Autodesk Inventor part; units mm, degrees
(part 4 of 4)
  spline S763 degree 2 poles (254.6918, 603.0222) (254.6054, 602.9877) (254.4448, 602.8889) (254.3954, 602.8543) knots 0 0 0 1 2 2 2
  line L811 (254.3954, 602.8543) -> (254.3732, 602.8543)
  line L812 (254.3732, 602.8543) -> (254.3732, 603.289)
  spline S764 degree 2 poles (254.3732, 603.289) (254.4991, 603.3508) (254.9512, 603.4718) (255.1537, 603.4718) knots 0 0 0 1 2 2 2
  spline S765 degree 2 poles (255.1537, 603.4718) (255.581, 603.4718) (256.0627, 603.0198) (256.0627, 602.6344) knots 0 0 0 1 2 2 2
  spline S766 degree 2 poles (256.0627, 602.6344) (256.0627, 602.4541) (255.9787, 602.1528) (255.9046, 602.0244) knots 0 0 0 1 2 2 2
  spline S767 degree 2 poles (255.9046, 602.0244) (255.8305, 601.891) (255.6156, 601.6292) (255.497, 601.5032) knots 0 0 0 1 2 2 2
  spline S768 degree 2 poles (255.497, 601.5032) (255.3044, 601.2932) (254.8326, 600.8437) (254.6918, 600.7128) knots 0 0 0 1 2 2 2
  line L813 (254.6918, 600.7128) -> (256.1886, 600.7128)
  line L814 (256.1886, 600.7128) -> (256.1886, 600.3596)
  line L815 (259.3305, 600.3596) -> (258.8068, 600.3596)
  line L816 (258.8068, 600.3596) -> (258.3894, 600.7968)
  spline S769 degree 2 poles (258.3894, 600.7968) (258.1819, 600.53) (257.7423, 600.2953) (257.4632, 600.2953) knots 0 0 0 1 2 2 2
  spline S770 degree 2 poles (257.4632, 600.2953) (257.0507, 600.2953) (256.5122, 600.7943) (256.5122, 601.1969) knots 0 0 0 1 2 2 2
  spline S771 degree 2 poles (256.5122, 601.1969) (256.5122, 601.3723) (256.611, 601.6464) (256.6925, 601.7576) knots 0 0 0 1 2 2 2
  spline S772 degree 2 poles (256.6925, 601.7576) (256.7716, 601.8638) (256.9815, 602.0268) (257.0754, 602.0861) knots 0 0 0 1 2 2 2
  spline S773 degree 2 poles (257.0754, 602.0861) (256.8704, 602.2244) (256.6653, 602.5332) (256.6653, 602.7654) knots 0 0 0 1 2 2 2
  spline S774 degree 2 poles (256.6653, 602.7654) (256.6653, 602.9111) (256.7814, 603.1581) (256.8753, 603.252) knots 0 0 0 1 2 2 2
  spline S775 degree 2 poles (256.8753, 603.252) (256.9741, 603.3483) (257.2878, 603.4718) (257.473, 603.4718) knots 0 0 0 1 2 2 2
  spline S776 degree 2 poles (257.473, 603.4718) (257.8139, 603.4718) (258.2437, 603.1136) (258.2437, 602.8395) knots 0 0 0 1 2 2 2
  spline S777 degree 2 poles (258.2437, 602.8395) (258.2437, 602.7382) (258.1918, 602.5233) (258.1251, 602.4245) knots 0 0 0 1 2 2 2
  spline S778 degree 2 poles (258.1251, 602.4245) (258.056, 602.3232) (257.8386, 602.1479) (257.6558, 602.0812) knots 0 0 0 1 2 2 2
  line L817 (257.6558, 602.0812) -> (258.3746, 601.3402)
  spline S779 degree 2 poles (258.3746, 601.3402) (258.4018, 601.5081) (258.4141, 601.9033) (258.4141, 602.222) knots 0 0 0 1 2 2 2
  line L818 (258.4141, 602.222) -> (258.8143, 602.222)
  line L819 (258.8143, 602.222) -> (258.8143, 602.0244)
  spline S780 degree 2 poles (258.8143, 602.0244) (258.8143, 601.8292) (258.7155, 601.3352) (258.5994, 601.1129) knots 0 0 0 1 2 2 2
  line L820 (258.5994, 601.1129) -> (259.3305, 600.3596)
  line L821 (258.2116, 600.9771) -> (257.2705, 601.9404)
  spline S781 degree 2 poles (257.2705, 601.9404) (257.2211, 601.9083) (257.1198, 601.8169) (257.0581, 601.728) knots 0 0 0 1 2 2 2
  spline S782 degree 2 poles (257.0581, 601.728) (257.0087, 601.6563) (256.9346, 601.4241) (256.9346, 601.2957) knots 0 0 0 1 2 2 2
  spline S783 degree 2 poles (256.9346, 601.2957) (256.9346, 601.0042) (257.2804, 600.6288) (257.5743, 600.6288) knots 0 0 0 1 2 2 2
  spline S784 degree 2 poles (257.5743, 600.6288) (257.7694, 600.6288) (258.0831, 600.7943) (258.2116, 600.9771) knots 0 0 0 1 2 2 2
  spline S785 degree 2 poles (257.4632, 602.2269) (257.5768, 602.2664) (257.7275, 602.3973) (257.7694, 602.4739) knots 0 0 0 1 2 2 2
  spline S786 degree 2 poles (257.7694, 602.4739) (257.8065, 602.5455) (257.8435, 602.7061) (257.8435, 602.7999) knots 0 0 0 1 2 2 2
  spline S787 degree 2 poles (257.8435, 602.7999) (257.8435, 602.9975) (257.6114, 603.2149) (257.4582, 603.2149) knots 0 0 0 1 2 2 2
  spline S788 degree 2 poles (257.4582, 603.2149) (257.2754, 603.2149) (257.0655, 602.9679) (257.0655, 602.7851) knots 0 0 0 1 2 2 2
  spline S789 degree 2 poles (257.0655, 602.7851) (257.0655, 602.7036) (257.0951, 602.585) (257.1445, 602.5085) knots 0 0 0 1 2 2 2
  spline S790 degree 2 poles (257.1445, 602.5085) (257.189, 602.4443) (257.3421, 602.301) (257.4632, 602.2269) knots 0 0 0 1 2 2 2
  spline S791 degree 2 poles (260.0937, 600.3052) (259.864, 600.3052) (259.4663, 600.4287) (259.3354, 600.4979) knots 0 0 0 1 2 2 2
  line L822 (259.3354, 600.4979) -> (259.3354, 600.9301)
  line L823 (259.3354, 600.9301) -> (259.3552, 600.9301)
  spline S792 degree 2 poles (259.3552, 600.9301) (259.4046, 600.8906) (259.538, 600.7968) (259.6491, 600.7449) knots 0 0 0 1 2 2 2
  spline S793 degree 2 poles (259.6491, 600.7449) (259.7455, 600.698) (259.9826, 600.6288) (260.1085, 600.6288) knots 0 0 0 1 2 2 2
  spline S794 degree 2 poles (260.1085, 600.6288) (260.1999, 600.6288) (260.4099, 600.6708) (260.4593, 600.7054) knots 0 0 0 1 2 2 2
  spline S795 degree 2 poles (260.4593, 600.7054) (260.5309, 600.7523) (260.5951, 600.8585) (260.5951, 600.9672) knots 0 0 0 1 2 2 2
  spline S796 degree 2 poles (260.5951, 600.9672) (260.5951, 601.103) (260.4469, 601.2438) (260.2567, 601.2908) knots 0 0 0 1 2 2 2
  spline S797 degree 2 poles (260.2567, 601.2908) (260.1826, 601.3081) (259.9455, 601.3575) (259.8443, 601.3846) knots 0 0 0 1 2 2 2
  spline S798 degree 2 poles (259.8443, 601.3846) (259.5824, 601.4612) (259.3453, 601.7774) (259.3453, 602.0021) knots 0 0 0 1 2 2 2
  spline S799 degree 2 poles (259.3453, 602.0021) (259.3453, 602.3133) (259.8121, 602.7011) (260.1975, 602.7011) knots 0 0 0 1 2 2 2
  spline S800 degree 2 poles (260.1975, 602.7011) (260.3877, 602.7011) (260.773, 602.6073) (260.9039, 602.5356) knots 0 0 0 1 2 2 2
  line L824 (260.9039, 602.5356) -> (260.9039, 602.1232)
  line L825 (260.9039, 602.1232) -> (260.8841, 602.1232)
  spline S801 degree 2 poles (260.8841, 602.1232) (260.7359, 602.2417) (260.3753, 602.3776) (260.1901, 602.3776) knots 0 0 0 1 2 2 2
  spline S802 degree 2 poles (260.1901, 602.3776) (259.9999, 602.3776) (259.738, 602.217) (259.738, 602.0565) knots 0 0 0 1 2 2 2
  spline S803 degree 2 poles (259.738, 602.0565) (259.738, 601.9107) (259.8937, 601.7699) (260.0666, 601.7255) knots 0 0 0 1 2 2 2
  spline S804 degree 2 poles (260.0666, 601.7255) (260.1505, 601.7033) (260.363, 601.6588) (260.479, 601.6316) knots 0 0 0 1 2 2 2
  spline S805 degree 2 poles (260.479, 601.6316) (260.731, 601.5674) (260.9879, 601.2735) (260.9879, 601.0191) knots 0 0 0 1 2 2 2
  spline S806 degree 2 poles (260.9879, 601.0191) (260.9879, 600.8709) (260.8718, 600.609) (260.7582, 600.5127) knots 0 0 0 1 2 2 2
  spline S807 degree 2 poles (260.7582, 600.5127) (260.6371, 600.4114) (260.3284, 600.3052) (260.0937, 600.3052) knots 0 0 0 1 2 2 2
  line L826 (262.5588, 602.2343) -> (262.539, 602.2343)
  spline S808 degree 2 poles (262.539, 602.2343) (262.4946, 602.2467) (262.3983, 602.2516) (262.3316, 602.2516) knots 0 0 0 1 2 2 2
  spline S809 degree 2 poles (262.3316, 602.2516) (262.176, 602.2516) (261.8697, 602.1157) (261.7313, 601.9824) knots 0 0 0 1 2 2 2
  line L827 (261.7313, 601.9824) -> (261.7313, 600.3596)
  line L828 (261.7313, 600.3596) -> (261.346, 600.3596)
  line L829 (261.346, 600.3596) -> (261.346, 602.6468)
  line L830 (261.346, 602.6468) -> (261.7313, 602.6468)
  line L831 (261.7313, 602.6468) -> (261.7313, 602.3059)
  spline S810 degree 2 poles (261.7313, 602.3059) (261.9413, 602.4937) (262.255, 602.6468) (262.4032, 602.6468) knots 0 0 0 1 2 2 2
  spline S811 degree 2 poles (262.4032, 602.6468) (262.4625, 602.6468) (262.5218, 602.6419) (262.5588, 602.6344) knots 0 0 0 1 2 2 2
  line L832 (262.5588, 602.6344) -> (262.5588, 602.2343)
  line L833 (265.2338, 601.1006) -> (262.9713, 601.1006)
  line L834 (262.9713, 601.1006) -> (262.9713, 601.4291)
  line L835 (262.9713, 601.4291) -> (265.2338, 601.4291)
  line L836 (265.2338, 601.4291) -> (265.2338, 601.1006)
  line L837 (265.2338, 601.9601) -> (262.9713, 601.9601)
  line L838 (262.9713, 601.9601) -> (262.9713, 602.2886)
  line L839 (262.9713, 602.2886) -> (265.2338, 602.2886)
  line L840 (265.2338, 602.2886) -> (265.2338, 601.9601)
  spline S812 degree 2 poles (266.7727, 600.2904) (266.5454, 600.2904) (266.1724, 600.4263) (266.0415, 600.5522) knots 0 0 0 1 2 2 2
  spline S813 degree 2 poles (266.0415, 600.5522) (265.9131, 600.6757) (265.7797, 601.0116) (265.7797, 601.2018) knots 0 0 0 1 2 2 2
  spline S814 degree 2 poles (265.7797, 601.2018) (265.7797, 601.4488) (266.044, 601.8638) (266.2959, 601.9873) knots 0 0 0 1 2 2 2
  line L841 (266.2959, 601.9873) -> (266.2959, 601.9997)
  spline S815 degree 2 poles (266.2959, 601.9997) (266.0712, 602.1306) (265.8538, 602.4418) (265.8538, 602.674) knots 0 0 0 1 2 2 2
  spline S816 degree 2 poles (265.8538, 602.674) (265.8538, 603.0173) (266.3725, 603.4767) (266.7727, 603.4767) knots 0 0 0 1 2 2 2
  spline S817 degree 2 poles (266.7727, 603.4767) (267.1876, 603.4767) (267.689, 603.042) (267.689, 602.7011) knots 0 0 0 1 2 2 2
  spline S818 degree 2 poles (267.689, 602.7011) (267.689, 602.4961) (267.4494, 602.096) (267.2247, 601.9824) knots 0 0 0 1 2 2 2
  line L842 (267.2247, 601.9824) -> (267.2247, 601.97)
  spline S819 degree 2 poles (267.2247, 601.97) (267.4914, 601.8465) (267.7656, 601.4908) (267.7656, 601.2093) knots 0 0 0 1 2 2 2
  spline S820 degree 2 poles (267.7656, 601.2093) (267.7656, 600.819) (267.1975, 600.2904) (266.7727, 600.2904) knots 0 0 0 1 2 2 2
  spline S821 degree 2 poles (267.3457, 601.1697) (267.3457, 601.3575) (267.1975, 601.5798) (266.9875, 601.6934) knots 0 0 0 1 2 2 2
  spline S822 degree 2 poles (266.9875, 601.6934) (266.9184, 601.7329) (266.6862, 601.8243) (266.5405, 601.8836) knots 0 0 0 1 2 2 2
  spline S823 degree 2 poles (266.5405, 601.8836) (266.3725, 601.7724) (266.1922, 601.4414) (266.1922, 601.2315) knots 0 0 0 1 2 2 2
  spline S824 degree 2 poles (266.1922, 601.2315) (266.1922, 600.9548) (266.5256, 600.5942) (266.7776, 600.5942) knots 0 0 0 1 2 2 2
  spline S825 degree 2 poles (266.7776, 600.5942) (267.0345, 600.5942) (267.3457, 600.903) (267.3457, 601.1697) knots 0 0 0 1 2 2 2
  spline S826 degree 2 poles (267.2889, 602.6962) (267.2889, 602.9012) (267.0147, 603.1754) (266.7702, 603.1754) knots 0 0 0 1 2 2 2
  spline S827 degree 2 poles (266.7702, 603.1754) (266.5479, 603.1754) (266.2638, 602.9309) (266.2638, 602.7209) knots 0 0 0 1 2 2 2
  spline S828 degree 2 poles (266.2638, 602.7209) (266.2638, 602.5702) (266.4096, 602.3603) (266.5553, 602.2763) knots 0 0 0 1 2 2 2
  spline S829 degree 2 poles (266.5553, 602.2763) (266.617, 602.2417) (266.8789, 602.1207) (266.9851, 602.0861) knots 0 0 0 1 2 2 2
  spline S830 degree 2 poles (266.9851, 602.0861) (267.1629, 602.222) (267.2889, 602.5109) (267.2889, 602.6962) knots 0 0 0 1 2 2 2
  line L843 (269.255, 601.5081) -> (268.1015, 601.5081)
  line L844 (268.1015, 601.5081) -> (268.1015, 601.8786)
  line L845 (268.1015, 601.8786) -> (269.255, 601.8786)
  line L846 (269.255, 601.8786) -> (269.255, 601.5081)
  spline S831 degree 2 poles (270.4826, 603.1186) (270.3715, 603.1186) (270.1516, 603.0642) (270.0454, 603.0222) knots 0 0 0 1 2 2 2
  spline S832 degree 2 poles (270.0454, 603.0222) (269.9466, 602.9803) (269.8009, 602.8913) (269.7441, 602.8518) knots 0 0 0 1 2 2 2
  line L847 (269.7441, 602.8518) -> (269.7194, 602.8518)
  line L848 (269.7194, 602.8518) -> (269.7194, 603.2841)
  spline S833 degree 2 poles (269.7194, 603.2841) (269.8528, 603.3557) (270.3097, 603.4718) (270.5147, 603.4718) knots 0 0 0 1 2 2 2
  spline S834 degree 2 poles (270.5147, 603.4718) (270.7222, 603.4718) (271.031, 603.3878) (271.1569, 603.2989) knots 0 0 0 1 2 2 2
  spline S835 degree 2 poles (271.1569, 603.2989) (271.2903, 603.2026) (271.4286, 602.9234) (271.4286, 602.7357) knots 0 0 0 1 2 2 2
  spline S836 degree 2 poles (271.4286, 602.7357) (271.4286, 602.4838) (271.0976, 602.1034) (270.8655, 602.054) knots 0 0 0 1 2 2 2
  line L849 (270.8655, 602.054) -> (270.8655, 602.0244)
  spline S837 degree 2 poles (270.8655, 602.0244) (270.9618, 602.0046) (271.1816, 601.9157) (271.2755, 601.8268) knots 0 0 0 1 2 2 2
  spline S838 degree 2 poles (271.2755, 601.8268) (271.3694, 601.7403) (271.4879, 601.4637) (271.4879, 601.2636) knots 0 0 0 1 2 2 2
  spline S839 degree 2 poles (271.4879, 601.2636) (271.4879, 601.0586) (271.3471, 600.7103) (271.2187, 600.5769) knots 0 0 0 1 2 2 2
  spline S840 degree 2 poles (271.2187, 600.5769) (271.0853, 600.4386) (270.7074, 600.2953) (270.4678, 600.2953) knots 0 0 0 1 2 2 2
  spline S841 degree 2 poles (270.4678, 600.2953) (270.2381, 600.2953) (269.7885, 600.4065) (269.6354, 600.4831) knots 0 0 0 1 2 2 2
  line L850 (269.6354, 600.4831) -> (269.6354, 600.9153)
  line L851 (269.6354, 600.9153) -> (269.665, 600.9153)
  spline S842 degree 2 poles (269.665, 600.9153) (269.7935, 600.8215) (270.2282, 600.6486) (270.4431, 600.6486) knots 0 0 0 1 2 2 2
  spline S843 degree 2 poles (270.4431, 600.6486) (270.5691, 600.6486) (270.821, 600.7276) (270.905, 600.819) knots 0 0 0 1 2 2 2
  spline S844 degree 2 poles (270.905, 600.819) (270.9865, 600.9104) (271.0729, 601.1277) (271.0729, 601.2932) knots 0 0 0 1 2 2 2
  spline S845 degree 2 poles (271.0729, 601.2932) (271.0729, 601.4587) (270.9766, 601.6736) (270.8902, 601.7354) knots 0 0 0 1 2 2 2
  spline S846 degree 2 poles (270.8902, 601.7354) (270.8037, 601.7971) (270.5691, 601.844) (270.4307, 601.844) knots 0 0 0 1 2 2 2
  line L852 (270.4307, 601.844) -> (270.2578, 601.844)
  line L853 (270.2578, 601.844) -> (270.2578, 602.1824)
  line L854 (270.2578, 602.1824) -> (270.3937, 602.1824)
  spline S847 degree 2 poles (270.3937, 602.1824) (270.6679, 602.1824) (271.0137, 602.4443) (271.0137, 602.6937) knots 0 0 0 1 2 2 2
  spline S848 degree 2 poles (271.0137, 602.6937) (271.0137, 602.8098) (270.9247, 602.9753) (270.8531, 603.0247) knots 0 0 0 1 2 2 2
  spline S849 degree 2 poles (270.8531, 603.0247) (270.7765, 603.0766) (270.5888, 603.1186) (270.4826, 603.1186) knots 0 0 0 1 2 2 2
  line L855 (274.6816, 600.3596) -> (274.158, 600.3596)
  line L856 (274.158, 600.3596) -> (273.7406, 600.7968)
  spline S850 degree 2 poles (273.7406, 600.7968) (273.5331, 600.53) (273.0934, 600.2953) (272.8143, 600.2953) knots 0 0 0 1 2 2 2
  spline S851 degree 2 poles (272.8143, 600.2953) (272.4018, 600.2953) (271.8634, 600.7943) (271.8634, 601.1969) knots 0 0 0 1 2 2 2
  spline S852 degree 2 poles (271.8634, 601.1969) (271.8634, 601.3723) (271.9622, 601.6464) (272.0437, 601.7576) knots 0 0 0 1 2 2 2
  spline S853 degree 2 poles (272.0437, 601.7576) (272.1227, 601.8638) (272.3327, 602.0268) (272.4265, 602.0861) knots 0 0 0 1 2 2 2
  spline S854 degree 2 poles (272.4265, 602.0861) (272.2215, 602.2244) (272.0165, 602.5332) (272.0165, 602.7654) knots 0 0 0 1 2 2 2
  spline S855 degree 2 poles (272.0165, 602.7654) (272.0165, 602.9111) (272.1326, 603.1581) (272.2264, 603.252) knots 0 0 0 1 2 2 2
  spline S856 degree 2 poles (272.2264, 603.252) (272.3252, 603.3483) (272.6389, 603.4718) (272.8242, 603.4718) knots 0 0 0 1 2 2 2
  spline S857 degree 2 poles (272.8242, 603.4718) (273.1651, 603.4718) (273.5948, 603.1136) (273.5948, 602.8395) knots 0 0 0 1 2 2 2
  spline S858 degree 2 poles (273.5948, 602.8395) (273.5948, 602.7382) (273.543, 602.5233) (273.4763, 602.4245) knots 0 0 0 1 2 2 2
  spline S859 degree 2 poles (273.4763, 602.4245) (273.4071, 602.3232) (273.1898, 602.1479) (273.007, 602.0812) knots 0 0 0 1 2 2 2
  line L857 (273.007, 602.0812) -> (273.7257, 601.3402)
  spline S860 degree 2 poles (273.7257, 601.3402) (273.7529, 601.5081) (273.7653, 601.9033) (273.7653, 602.222) knots 0 0 0 1 2 2 2
  line L858 (273.7653, 602.222) -> (274.1654, 602.222)
  line L859 (274.1654, 602.222) -> (274.1654, 602.0244)
  spline S861 degree 2 poles (274.1654, 602.0244) (274.1654, 601.8292) (274.0666, 601.3352) (273.9505, 601.1129) knots 0 0 0 1 2 2 2
  line L860 (273.9505, 601.1129) -> (274.6816, 600.3596)
  line L861 (273.5627, 600.9771) -> (272.6216, 601.9404)
  spline S862 degree 2 poles (272.6216, 601.9404) (272.5722, 601.9083) (272.471, 601.8169) (272.4092, 601.728) knots 0 0 0 1 2 2 2
  spline S863 degree 2 poles (272.4092, 601.728) (272.3598, 601.6563) (272.2857, 601.4241) (272.2857, 601.2957) knots 0 0 0 1 2 2 2
  spline S864 degree 2 poles (272.2857, 601.2957) (272.2857, 601.0042) (272.6315, 600.6288) (272.9255, 600.6288) knots 0 0 0 1 2 2 2
  spline S865 degree 2 poles (272.9255, 600.6288) (273.1206, 600.6288) (273.4343, 600.7943) (273.5627, 600.9771) knots 0 0 0 1 2 2 2
  spline S866 degree 2 poles (272.8143, 602.2269) (272.9279, 602.2664) (273.0786, 602.3973) (273.1206, 602.4739) knots 0 0 0 1 2 2 2
  spline S867 degree 2 poles (273.1206, 602.4739) (273.1576, 602.5455) (273.1947, 602.7061) (273.1947, 602.7999) knots 0 0 0 1 2 2 2
  spline S868 degree 2 poles (273.1947, 602.7999) (273.1947, 602.9975) (272.9625, 603.2149) (272.8094, 603.2149) knots 0 0 0 1 2 2 2
  spline S869 degree 2 poles (272.8094, 603.2149) (272.6266, 603.2149) (272.4166, 602.9679) (272.4166, 602.7851) knots 0 0 0 1 2 2 2
  spline S870 degree 2 poles (272.4166, 602.7851) (272.4166, 602.7036) (272.4463, 602.585) (272.4957, 602.5085) knots 0 0 0 1 2 2 2
  spline S871 degree 2 poles (272.4957, 602.5085) (272.5401, 602.4443) (272.6933, 602.301) (272.8143, 602.2269) knots 0 0 0 1 2 2 2
  line L862 (276.7219, 600.3596) -> (276.2155, 600.3596)
  line L863 (276.2155, 600.3596) -> (275.3658, 601.4637)
  line L864 (275.3658, 601.4637) -> (275.2127, 601.3155)
  line L865 (275.2127, 601.3155) -> (275.2127, 600.3596)
  line L866 (275.2127, 600.3596) -> (274.8274, 600.3596)
  line L867 (274.8274, 600.3596) -> (274.8274, 603.5434)
  line L868 (274.8274, 603.5434) -> (275.2127, 603.5434)
  line L869 (275.2127, 603.5434) -> (275.2127, 601.681)
  line L870 (275.2127, 601.681) -> (276.1167, 602.6468)
  line L871 (276.1167, 602.6468) -> (276.5959, 602.6468)
  line L872 (276.5959, 602.6468) -> (275.6573, 601.6909)
  line L873 (275.6573, 601.6909) -> (276.7219, 600.3596)
  spline S872 degree 2 poles (277.9075, 600.3077) (277.3591, 600.3077) (276.7565, 600.9227) (276.7565, 601.4908) knots 0 0 0 1 2 2 2
  spline S873 degree 2 poles (276.7565, 601.4908) (276.7565, 602.0491) (277.3418, 602.711) (277.8136, 602.711) knots 0 0 0 1 2 2 2
  spline S874 degree 2 poles (277.8136, 602.711) (278.026, 602.711) (278.3546, 602.5875) (278.4756, 602.4566) knots 0 0 0 1 2 2 2
  spline S875 degree 2 poles (278.4756, 602.4566) (278.5991, 602.3257) (278.73, 601.9478) (278.73, 601.6736) knots 0 0 0 1 2 2 2
  line L874 (278.73, 601.6736) -> (278.73, 601.4637)
  line L875 (278.73, 601.4637) -> (277.1467, 601.4637)
  spline S876 degree 2 poles (277.1467, 601.4637) (277.1467, 601.066) (277.5469, 600.6436) (277.9025, 600.6436) knots 0 0 0 1 2 2 2
  spline S877 degree 2 poles (277.9025, 600.6436) (278.0285, 600.6436) (278.273, 600.7004) (278.3718, 600.7449) knots 0 0 0 1 2 2 2
  spline S878 degree 2 poles (278.3718, 600.7449) (278.4756, 600.7943) (278.6188, 600.8807) (278.6658, 600.9203) knots 0 0 0 1 2 2 2
  line L876 (278.6658, 600.9203) -> (278.688, 600.9203)
  line L877 (278.688, 600.9203) -> (278.688, 600.5004)
  spline S879 degree 2 poles (278.688, 600.5004) (278.6213, 600.4732) (278.4188, 600.3941) (278.3397, 600.3719) knots 0 0 0 1 2 2 2
  spline S880 degree 2 poles (278.3397, 600.3719) (278.2286, 600.3398) (278.0458, 600.3077) (277.9075, 600.3077) knots 0 0 0 1 2 2 2
  spline S881 degree 2 poles (278.3546, 601.7576) (278.3496, 601.9132) (278.2854, 602.1404) (278.2236, 602.217) knots 0 0 0 1 2 2 2
  spline S882 degree 2 poles (278.2236, 602.217) (278.157, 602.3035) (277.947, 602.3949) (277.7914, 602.3949) knots 0 0 0 1 2 2 2
  spline S883 degree 2 poles (277.7914, 602.3949) (277.6383, 602.3949) (277.4234, 602.3035) (277.3344, 602.2145) knots 0 0 0 1 2 2 2
  spline S884 degree 2 poles (277.3344, 602.2145) (277.248, 602.1232) (277.1591, 601.9033) (277.1467, 601.7576) knots 0 0 0 1 2 2 2
  line L878 (277.1467, 601.7576) -> (278.3546, 601.7576)
  line L879 (280.916, 602.6468) -> (279.6859, 599.5173)
  line L880 (279.6859, 599.5173) -> (279.2734, 599.5173)
  line L881 (279.2734, 599.5173) -> (279.6834, 600.4707)
  line L882 (279.6834, 600.4707) -> (278.8535, 602.6468)
  line L883 (278.8535, 602.6468) -> (279.2685, 602.6468)
  line L884 (279.2685, 602.6468) -> (279.8934, 600.9524)
  line L885 (279.8934, 600.9524) -> (280.5158, 602.6468)
  line L886 (280.5158, 602.6468) -> (280.916, 602.6468)
  line L887 (283.9788, 602.6468) -> (283.3983, 600.3596)
  line L888 (283.3983, 600.3596) -> (283.0426, 600.3596)
  line L889 (283.0426, 600.3596) -> (282.4844, 602.1232)
  line L890 (282.4844, 602.1232) -> (281.9287, 600.3596)
  line L891 (281.9287, 600.3596) -> (281.5755, 600.3596)
  line L892 (281.5755, 600.3596) -> (280.9901, 602.6468)
  line L893 (280.9901, 602.6468) -> (281.3902, 602.6468)
  line L894 (281.3902, 602.6468) -> (281.7953, 600.8758)
  line L895 (281.7953, 600.8758) -> (282.3362, 602.6468)
  line L896 (282.3362, 602.6468) -> (282.6549, 602.6468)
  line L897 (282.6549, 602.6468) -> (283.2106, 600.8758)
  line L898 (283.2106, 600.8758) -> (283.591, 602.6468)
  line L899 (283.591, 602.6468) -> (283.9788, 602.6468)
  spline S885 degree 2 poles (286.1969, 601.5032) (286.1969, 600.9252) (285.6411, 600.2953) (285.1767, 600.2953) knots 0 0 0 1 2 2 2
  spline S886 degree 2 poles (285.1767, 600.2953) (284.7, 600.2953) (284.1542, 600.945) (284.1542, 601.5032) knots 0 0 0 1 2 2 2
  spline S887 degree 2 poles (284.1542, 601.5032) (284.1542, 602.0762) (284.7173, 602.711) (285.1767, 602.711) knots 0 0 0 1 2 2 2
  spline S888 degree 2 poles (285.1767, 602.711) (285.6411, 602.711) (286.1969, 602.0787) (286.1969, 601.5032) knots 0 0 0 1 2 2 2
  spline S889 degree 2 poles (285.7992, 601.5032) (285.7992, 601.9478) (285.4756, 602.38) (285.1767, 602.38) knots 0 0 0 1 2 2 2
  spline S890 degree 2 poles (285.1767, 602.38) (284.8779, 602.38) (284.5518, 601.9478) (284.5518, 601.5032) knots 0 0 0 1 2 2 2
  spline S891 degree 2 poles (284.5518, 601.5032) (284.5518, 601.0709) (284.8779, 600.6263) (285.1767, 600.6263) knots 0 0 0 1 2 2 2
  spline S892 degree 2 poles (285.1767, 600.6263) (285.4731, 600.6263) (285.7992, 601.0635) (285.7992, 601.5032) knots 0 0 0 1 2 2 2
  line L900 (287.8048, 602.2343) -> (287.7851, 602.2343)
  spline S893 degree 2 poles (287.7851, 602.2343) (287.7406, 602.2467) (287.6443, 602.2516) (287.5776, 602.2516) knots 0 0 0 1 2 2 2
  spline S894 degree 2 poles (287.5776, 602.2516) (287.422, 602.2516) (287.1157, 602.1157) (286.9774, 601.9824) knots 0 0 0 1 2 2 2
  line L901 (286.9774, 601.9824) -> (286.9774, 600.3596)
  line L902 (286.9774, 600.3596) -> (286.5921, 600.3596)
  line L903 (286.5921, 600.3596) -> (286.5921, 602.6468)
  line L904 (286.5921, 602.6468) -> (286.9774, 602.6468)
  line L905 (286.9774, 602.6468) -> (286.9774, 602.3059)
  spline S895 degree 2 poles (286.9774, 602.3059) (287.1873, 602.4937) (287.501, 602.6468) (287.6492, 602.6468) knots 0 0 0 1 2 2 2
  spline S896 degree 2 poles (287.6492, 602.6468) (287.7085, 602.6468) (287.7678, 602.6419) (287.8048, 602.6344) knots 0 0 0 1 2 2 2
  line L906 (287.8048, 602.6344) -> (287.8048, 602.2343)
  line L907 (289.8624, 600.3596) -> (289.477, 600.3596)
  line L908 (289.477, 600.3596) -> (289.477, 600.5917)
  spline S897 degree 2 poles (289.477, 600.5917) (289.3881, 600.5176) (289.2572, 600.4188) (289.1683, 600.3769) knots 0 0 0 1 2 2 2
  spline S898 degree 2 poles (289.1683, 600.3769) (289.0868, 600.3373) (288.9114, 600.2953) (288.7953, 600.2953) knots 0 0 0 1 2 2 2
  spline S899 degree 2 poles (288.7953, 600.2953) (288.6076, 600.2953) (288.2914, 600.451) (288.1803, 600.6016) knots 0 0 0 1 2 2 2
  spline S900 degree 2 poles (288.1803, 600.6016) (288.0691, 600.7523) (287.9456, 601.1969) (287.9456, 601.4859) knots 0 0 0 1 2 2 2
  spline S901 degree 2 poles (287.9456, 601.4859) (287.9456, 601.7872) (288.1012, 602.2269) (288.2371, 602.3924) knots 0 0 0 1 2 2 2
  spline S902 degree 2 poles (288.2371, 602.3924) (288.3631, 602.5406) (288.7163, 602.711) (288.9114, 602.711) knots 0 0 0 1 2 2 2
  spline S903 degree 2 poles (288.9114, 602.711) (289.0818, 602.711) (289.3362, 602.6344) (289.477, 602.5554) knots 0 0 0 1 2 2 2
  line L909 (289.477, 602.5554) -> (289.477, 603.5434)
  line L910 (289.477, 603.5434) -> (289.8624, 603.5434)
  line L911 (289.8624, 603.5434) -> (289.8624, 600.3596)
  line L912 (289.477, 600.9153) -> (289.477, 602.2368)
  spline S904 degree 2 poles (289.477, 602.2368) (289.3338, 602.3059) (289.1065, 602.3578) (288.9756, 602.3578) knots 0 0 0 1 2 2 2
  spline S905 degree 2 poles (288.9756, 602.3578) (288.6792, 602.3578) (288.3433, 601.9132) (288.3433, 601.4933) knots 0 0 0 1 2 2 2
  spline S906 degree 2 poles (288.3433, 601.4933) (288.3433, 601.0882) (288.6002, 600.6609) (288.8842, 600.6609) knots 0 0 0 1 2 2 2
  spline S907 degree 2 poles (288.8842, 600.6609) (289.0349, 600.6609) (289.3412, 600.7992) (289.477, 600.9153) knots 0 0 0 1 2 2 2
  spline S908 degree 2 poles (291.0381, 600.3052) (290.8084, 600.3052) (290.4107, 600.4287) (290.2798, 600.4979) knots 0 0 0 1 2 2 2
  line L913 (290.2798, 600.4979) -> (290.2798, 600.9301)
  line L914 (290.2798, 600.9301) -> (290.2996, 600.9301)
  spline S909 degree 2 poles (290.2996, 600.9301) (290.349, 600.8906) (290.4823, 600.7968) (290.5935, 600.7449) knots 0 0 0 1 2 2 2
  spline S910 degree 2 poles (290.5935, 600.7449) (290.6898, 600.698) (290.9269, 600.6288) (291.0529, 600.6288) knots 0 0 0 1 2 2 2
  spline S911 degree 2 poles (291.0529, 600.6288) (291.1443, 600.6288) (291.3543, 600.6708) (291.4037, 600.7054) knots 0 0 0 1 2 2 2
  spline S912 degree 2 poles (291.4037, 600.7054) (291.4753, 600.7523) (291.5395, 600.8585) (291.5395, 600.9672) knots 0 0 0 1 2 2 2
  spline S913 degree 2 poles (291.5395, 600.9672) (291.5395, 601.103) (291.3913, 601.2438) (291.2011, 601.2908) knots 0 0 0 1 2 2 2
  spline S914 degree 2 poles (291.2011, 601.2908) (291.127, 601.3081) (290.8899, 601.3575) (290.7886, 601.3846) knots 0 0 0 1 2 2 2
  spline S915 degree 2 poles (290.7886, 601.3846) (290.5268, 601.4612) (290.2897, 601.7774) (290.2897, 602.0021) knots 0 0 0 1 2 2 2
  spline S916 degree 2 poles (290.2897, 602.0021) (290.2897, 602.3133) (290.7565, 602.7011) (291.1418, 602.7011) knots 0 0 0 1 2 2 2
  spline S917 degree 2 poles (291.1418, 602.7011) (291.332, 602.7011) (291.7173, 602.6073) (291.8483, 602.5356) knots 0 0 0 1 2 2 2
  line L915 (291.8483, 602.5356) -> (291.8483, 602.1232)
  line L916 (291.8483, 602.1232) -> (291.8285, 602.1232)
  spline S918 degree 2 poles (291.8285, 602.1232) (291.6803, 602.2417) (291.3197, 602.3776) (291.1344, 602.3776) knots 0 0 0 1 2 2 2
  spline S919 degree 2 poles (291.1344, 602.3776) (290.9442, 602.3776) (290.6824, 602.217) (290.6824, 602.0565) knots 0 0 0 1 2 2 2
  spline S920 degree 2 poles (290.6824, 602.0565) (290.6824, 601.9107) (290.838, 601.7699) (291.0109, 601.7255) knots 0 0 0 1 2 2 2
  spline S921 degree 2 poles (291.0109, 601.7255) (291.0949, 601.7033) (291.3073, 601.6588) (291.4234, 601.6316) knots 0 0 0 1 2 2 2
  spline S922 degree 2 poles (291.4234, 601.6316) (291.6754, 601.5674) (291.9322, 601.2735) (291.9322, 601.0191) knots 0 0 0 1 2 2 2
  spline S923 degree 2 poles (291.9322, 601.0191) (291.9322, 600.8709) (291.8161, 600.609) (291.7025, 600.5127) knots 0 0 0 1 2 2 2
  spline S924 degree 2 poles (291.7025, 600.5127) (291.5815, 600.4114) (291.2727, 600.3052) (291.0381, 600.3052) knots 0 0 0 1 2 2 2
  line L917 (294.6665, 601.1006) -> (292.404, 601.1006)
  line L918 (292.404, 601.1006) -> (292.404, 601.4291)
  line L919 (292.404, 601.4291) -> (294.6665, 601.4291)
  line L920 (294.6665, 601.4291) -> (294.6665, 601.1006)
  line L921 (294.6665, 601.9601) -> (292.404, 601.9601)
  line L922 (292.404, 601.9601) -> (292.404, 602.2886)
  line L923 (292.404, 602.2886) -> (294.6665, 602.2886)
  line L924 (294.6665, 602.2886) -> (294.6665, 601.9601)
  line L925 (297.0995, 600.3596) -> (296.7142, 600.3596)
  line L926 (296.7142, 600.3596) -> (296.7142, 600.5917)
  spline S925 degree 2 poles (296.7142, 600.5917) (296.6253, 600.5176) (296.4944, 600.4188) (296.4054, 600.3769) knots 0 0 0 1 2 2 2
  spline S926 degree 2 poles (296.4054, 600.3769) (296.3239, 600.3373) (296.1486, 600.2953) (296.0325, 600.2953) knots 0 0 0 1 2 2 2
  spline S927 degree 2 poles (296.0325, 600.2953) (295.8447, 600.2953) (295.5286, 600.451) (295.4174, 600.6016) knots 0 0 0 1 2 2 2
  spline S928 degree 2 poles (295.4174, 600.6016) (295.3063, 600.7523) (295.1828, 601.1969) (295.1828, 601.4859) knots 0 0 0 1 2 2 2
  spline S929 degree 2 poles (295.1828, 601.4859) (295.1828, 601.7872) (295.3384, 602.2269) (295.4742, 602.3924) knots 0 0 0 1 2 2 2
  spline S930 degree 2 poles (295.4742, 602.3924) (295.6002, 602.5406) (295.9534, 602.711) (296.1486, 602.711) knots 0 0 0 1 2 2 2
  spline S931 degree 2 poles (296.1486, 602.711) (296.319, 602.711) (296.5734, 602.6344) (296.7142, 602.5554) knots 0 0 0 1 2 2 2
  line L927 (296.7142, 602.5554) -> (296.7142, 603.5434)
  line L928 (296.7142, 603.5434) -> (297.0995, 603.5434)
  line L929 (297.0995, 603.5434) -> (297.0995, 600.3596)
  line L930 (296.7142, 600.9153) -> (296.7142, 602.2368)
  spline S932 degree 2 poles (296.7142, 602.2368) (296.5709, 602.3059) (296.3437, 602.3578) (296.2128, 602.3578) knots 0 0 0 1 2 2 2
  spline S933 degree 2 poles (296.2128, 602.3578) (295.9164, 602.3578) (295.5804, 601.9132) (295.5804, 601.4933) knots 0 0 0 1 2 2 2
  spline S934 degree 2 poles (295.5804, 601.4933) (295.5804, 601.0882) (295.8373, 600.6609) (296.1214, 600.6609) knots 0 0 0 1 2 2 2
  spline S935 degree 2 poles (296.1214, 600.6609) (296.2721, 600.6609) (296.5783, 600.7992) (296.7142, 600.9153) knots 0 0 0 1 2 2 2
  line L931 (298.8705, 602.2343) -> (298.8508, 602.2343)
  spline S936 degree 2 poles (298.8508, 602.2343) (298.8063, 602.2467) (298.71, 602.2516) (298.6433, 602.2516) knots 0 0 0 1 2 2 2
  spline S937 degree 2 poles (298.6433, 602.2516) (298.4877, 602.2516) (298.1814, 602.1157) (298.0431, 601.9824) knots 0 0 0 1 2 2 2
  line L932 (298.0431, 601.9824) -> (298.0431, 600.3596)
  line L933 (298.0431, 600.3596) -> (297.6577, 600.3596)
  line L934 (297.6577, 600.3596) -> (297.6577, 602.6468)
  line L935 (297.6577, 602.6468) -> (298.0431, 602.6468)
  line L936 (298.0431, 602.6468) -> (298.0431, 602.3059)
  spline S938 degree 2 poles (298.0431, 602.3059) (298.253, 602.4937) (298.5667, 602.6468) (298.7149, 602.6468) knots 0 0 0 1 2 2 2
  spline S939 degree 2 poles (298.7149, 602.6468) (298.7742, 602.6468) (298.8335, 602.6419) (298.8705, 602.6344) knots 0 0 0 1 2 2 2
  line L937 (298.8705, 602.6344) -> (298.8705, 602.2343)
  line L938 (300.9478, 600.3596) -> (300.5625, 600.3596)
  line L939 (300.5625, 600.3596) -> (300.5625, 600.6115)
  spline S940 degree 2 poles (300.5625, 600.6115) (300.3846, 600.4559) (300.066, 600.2953) (299.8684, 600.2953) knots 0 0 0 1 2 2 2
  spline S941 degree 2 poles (299.8684, 600.2953) (299.7202, 600.2953) (299.4559, 600.3941) (299.3596, 600.5004) knots 0 0 0 1 2 2 2
  spline S942 degree 2 poles (299.3596, 600.5004) (299.2608, 600.6066) (299.1521, 600.9301) (299.1521, 601.1623) knots 0 0 0 1 2 2 2
  line L940 (299.1521, 601.1623) -> (299.1521, 602.6468)
  line L941 (299.1521, 602.6468) -> (299.5374, 602.6468)
  line L942 (299.5374, 602.6468) -> (299.5374, 601.3426)
  spline S943 degree 2 poles (299.5374, 601.3426) (299.5374, 601.1598) (299.5646, 600.9203) (299.6115, 600.8313) knots 0 0 0 1 2 2 2
  spline S944 degree 2 poles (299.6115, 600.8313) (299.6584, 600.7424) (299.819, 600.6609) (299.9697, 600.6609) knots 0 0 0 1 2 2 2
  spline S945 degree 2 poles (299.9697, 600.6609) (300.1105, 600.6609) (300.4291, 600.8215) (300.5625, 600.9375) knots 0 0 0 1 2 2 2
  line L943 (300.5625, 600.9375) -> (300.5625, 602.6468)
  line L944 (300.5625, 602.6468) -> (300.9478, 602.6468)
  line L945 (300.9478, 602.6468) -> (300.9478, 600.3596)
  line L946 (304.0995, 600.3596) -> (304.0995, 601.6835)
  spline S946 degree 2 poles (304.0995, 601.6835) (304.0995, 601.8416) (304.0748, 602.1108) (304.0353, 602.1849) knots 0 0 0 1 2 2 2
  spline S947 degree 2 poles (304.0353, 602.1849) (303.9958, 602.2664) (303.8451, 602.3455) (303.7142, 602.3455) knots 0 0 0 1 2 2 2
  spline S948 degree 2 poles (303.7142, 602.3455) (303.5957, 602.3455) (303.324, 602.1997) (303.1807, 602.0614) knots 0 0 0 1 2 2 2
  spline S949 degree 2 poles (303.1807, 602.0614) (303.1832, 602.0268) (303.1881, 601.9305) (303.1881, 601.8663) knots 0 0 0 1 2 2 2
  line L947 (303.1881, 601.8663) -> (303.1881, 600.3596)
  line L948 (303.1881, 600.3596) -> (302.8028, 600.3596)
  line L949 (302.8028, 600.3596) -> (302.8028, 601.6835)
  spline S950 degree 2 poles (302.8028, 601.6835) (302.8028, 601.8416) (302.7781, 602.1108) (302.7386, 602.1849) knots 0 0 0 1 2 2 2
  spline S951 degree 2 poles (302.7386, 602.1849) (302.699, 602.2664) (302.5484, 602.3455) (302.4175, 602.3455) knots 0 0 0 1 2 2 2
  spline S952 degree 2 poles (302.4175, 602.3455) (302.294, 602.3455) (302.0198, 602.1898) (301.8913, 602.0688) knots 0 0 0 1 2 2 2
  line L950 (301.8913, 602.0688) -> (301.8913, 600.3596)
  line L951 (301.8913, 600.3596) -> (301.506, 600.3596)
  line L952 (301.506, 600.3596) -> (301.506, 602.6468)
  line L953 (301.506, 602.6468) -> (301.8913, 602.6468)
  line L954 (301.8913, 602.6468) -> (301.8913, 602.3949)
  spline S953 degree 2 poles (301.8913, 602.3949) (302.042, 602.5455) (302.3384, 602.711) (302.5163, 602.711) knots 0 0 0 1 2 2 2
  spline S954 degree 2 poles (302.5163, 602.711) (302.7188, 602.711) (303.0325, 602.5258) (303.114, 602.3158) knots 0 0 0 1 2 2 2
  spline S955 degree 2 poles (303.114, 602.3158) (303.2894, 602.5109) (303.6204, 602.711) (303.813, 602.711) knots 0 0 0 1 2 2 2
  spline S956 degree 2 poles (303.813, 602.711) (303.9612, 602.711) (304.2033, 602.6196) (304.2922, 602.5159) knots 0 0 0 1 2 2 2
  spline S957 degree 2 poles (304.2922, 602.5159) (304.3836, 602.4121) (304.4849, 602.1009) (304.4849, 601.8663) knots 0 0 0 1 2 2 2
  line L955 (304.4849, 601.8663) -> (304.4849, 600.3596)
  line L956 (304.4849, 600.3596) -> (304.0995, 600.3596)
  line L957 (307.476, 601.5304) -> (306.4436, 601.5304)
  line L958 (306.4436, 601.5304) -> (306.4436, 600.4979)
  line L959 (306.4436, 600.4979) -> (306.1027, 600.4979)
  line L960 (306.1027, 600.4979) -> (306.1027, 601.5304)
  line L961 (306.1027, 601.5304) -> (305.0703, 601.5304)
  line L962 (305.0703, 601.5304) -> (305.0703, 601.8589)
  line L963 (305.0703, 601.8589) -> (306.1027, 601.8589)
  line L964 (306.1027, 601.8589) -> (306.1027, 602.8913)
  line L965 (306.1027, 602.8913) -> (306.4436, 602.8913)
  line L966 (306.4436, 602.8913) -> (306.4436, 601.8589)
  line L967 (306.4436, 601.8589) -> (307.476, 601.8589)
  line L968 (307.476, 601.8589) -> (307.476, 601.5304)
  line L969 (309.872, 600.3596) -> (309.4866, 600.3596)
  line L970 (309.4866, 600.3596) -> (309.4866, 601.6637)
  spline S958 degree 2 poles (309.4866, 601.6637) (309.4866, 601.8218) (309.457, 602.0935) (309.4125, 602.175) knots 0 0 0 1 2 2 2
  spline S959 degree 2 poles (309.4125, 602.175) (309.3656, 602.2615) (309.1976, 602.3455) (309.0544, 602.3455) knots 0 0 0 1 2 2 2
  spline S960 degree 2 poles (309.0544, 602.3455) (308.9111, 602.3455) (308.6073, 602.1923) (308.4616, 602.0688) knots 0 0 0 1 2 2 2
  line L971 (308.4616, 602.0688) -> (308.4616, 600.3596)
  line L972 (308.4616, 600.3596) -> (308.0763, 600.3596)
  line L973 (308.0763, 600.3596) -> (308.0763, 603.5434)
  line L974 (308.0763, 603.5434) -> (308.4616, 603.5434)
  line L975 (308.4616, 603.5434) -> (308.4616, 602.3924)
  spline S961 degree 2 poles (308.4616, 602.3924) (308.6345, 602.548) (308.9679, 602.711) (309.1557, 602.711) knots 0 0 0 1 2 2 2
  spline S962 degree 2 poles (309.1557, 602.711) (309.4916, 602.711) (309.872, 602.2664) (309.872, 601.844) knots 0 0 0 1 2 2 2
  line L976 (309.872, 601.844) -> (309.872, 600.3596)
  spline S963 degree 2 poles (311.6874, 600.6016) (311.6405, 600.567) (311.4824, 600.4435) (311.4083, 600.4065) knots 0 0 0 1 2 2 2
  spline S964 degree 2 poles (311.4083, 600.4065) (311.307, 600.3522) (311.1169, 600.2953) (310.944, 600.2953) knots 0 0 0 1 2 2 2
  spline S965 degree 2 poles (310.944, 600.2953) (310.8032, 600.2953) (310.5487, 600.4016) (310.4524, 600.4979) knots 0 0 0 1 2 2 2
  spline S966 degree 2 poles (310.4524, 600.4979) (310.361, 600.5917) (310.2499, 600.8684) (310.2499, 601.0215) knots 0 0 0 1 2 2 2
  spline S967 degree 2 poles (310.2499, 601.0215) (310.2499, 601.2587) (310.4499, 601.5946) (310.6673, 601.6909) knots 0 0 0 1 2 2 2
  spline S968 degree 2 poles (310.6673, 601.6909) (310.86, 601.7798) (311.3836, 601.8465) (311.6874, 601.8638) knots 0 0 0 1 2 2 2
  line L977 (311.6874, 601.8638) -> (311.6874, 601.9379)
  spline S969 degree 2 poles (311.6874, 601.9379) (311.6874, 602.0713) (311.6059, 602.2368) (311.5318, 602.2837) knots 0 0 0 1 2 2 2
  spline S970 degree 2 poles (311.5318, 602.2837) (311.4577, 602.3306) (311.2453, 602.3603) (311.1317, 602.3603) knots 0 0 0 1 2 2 2
  spline S971 degree 2 poles (311.1317, 602.3603) (310.9983, 602.3603) (310.6377, 602.2812) (310.4574, 602.2047) knots 0 0 0 1 2 2 2
  line L978 (310.4574, 602.2047) -> (310.4351, 602.2047)
  line L979 (310.4351, 602.2047) -> (310.4351, 602.5974)
  spline S972 degree 2 poles (310.4351, 602.5974) (310.5413, 602.627) (310.939, 602.7011) (311.1341, 602.7011) knots 0 0 0 1 2 2 2
  spline S973 degree 2 poles (311.1341, 602.7011) (311.3713, 602.7011) (311.6948, 602.627) (311.8233, 602.5307) knots 0 0 0 1 2 2 2
  spline S974 degree 2 poles (311.8233, 602.5307) (311.9492, 602.4368) (312.0727, 602.138) (312.0727, 601.9231) knots 0 0 0 1 2 2 2
  line L980 (312.0727, 601.9231) -> (312.0727, 600.3596)
  line L981 (312.0727, 600.3596) -> (311.6874, 600.3596)
  line L982 (311.6874, 600.3596) -> (311.6874, 600.6016)
  line L983 (311.6874, 600.9227) -> (311.6874, 601.5575)
  spline S975 degree 2 poles (311.6874, 601.5575) (311.5491, 601.5452) (311.1317, 601.5032) (311.0008, 601.4637) knots 0 0 0 1 2 2 2
  spline S976 degree 2 poles (311.0008, 601.4637) (310.8476, 601.4167) (310.6475, 601.2216) (310.6475, 601.0487) knots 0 0 0 1 2 2 2
  spline S977 degree 2 poles (310.6475, 601.0487) (310.6475, 600.8511) (310.8699, 600.651) (311.0823, 600.651) knots 0 0 0 1 2 2 2
  spline S978 degree 2 poles (311.0823, 600.651) (311.2626, 600.651) (311.559, 600.8066) (311.6874, 600.9227) knots 0 0 0 1 2 2 2
  line L984 (313.8265, 602.2343) -> (313.8067, 602.2343)
  spline S979 degree 2 poles (313.8067, 602.2343) (313.7622, 602.2467) (313.6659, 602.2516) (313.5992, 602.2516) knots 0 0 0 1 2 2 2
  spline S980 degree 2 poles (313.5992, 602.2516) (313.4436, 602.2516) (313.1373, 602.1157) (312.999, 601.9824) knots 0 0 0 1 2 2 2
  line L985 (312.999, 601.9824) -> (312.999, 600.3596)
  line L986 (312.999, 600.3596) -> (312.6137, 600.3596)
  line L987 (312.6137, 600.3596) -> (312.6137, 602.6468)
  line L988 (312.6137, 602.6468) -> (312.999, 602.6468)
  line L989 (312.999, 602.6468) -> (312.999, 602.3059)
  spline S981 degree 2 poles (312.999, 602.3059) (313.209, 602.4937) (313.5226, 602.6468) (313.6708, 602.6468) knots 0 0 0 1 2 2 2
  spline S982 degree 2 poles (313.6708, 602.6468) (313.7301, 602.6468) (313.7894, 602.6419) (313.8265, 602.6344) knots 0 0 0 1 2 2 2
  line L990 (313.8265, 602.6344) -> (313.8265, 602.2343)
  line L991 (315.921, 600.3596) -> (315.5357, 600.3596)
  line L992 (315.5357, 600.3596) -> (315.5357, 601.6637)
  spline S983 degree 2 poles (315.5357, 601.6637) (315.5357, 601.8218) (315.5061, 602.0935) (315.4616, 602.175) knots 0 0 0 1 2 2 2
  spline S984 degree 2 poles (315.4616, 602.175) (315.4147, 602.2615) (315.2467, 602.3455) (315.1035, 602.3455) knots 0 0 0 1 2 2 2
  spline S985 degree 2 poles (315.1035, 602.3455) (314.9602, 602.3455) (314.6564, 602.1923) (314.5107, 602.0688) knots 0 0 0 1 2 2 2
  line L993 (314.5107, 602.0688) -> (314.5107, 600.3596)
  line L994 (314.5107, 600.3596) -> (314.1253, 600.3596)
  line L995 (314.1253, 600.3596) -> (314.1253, 602.6468)
  line L996 (314.1253, 602.6468) -> (314.5107, 602.6468)
  line L997 (314.5107, 602.6468) -> (314.5107, 602.3924)
  spline S986 degree 2 poles (314.5107, 602.3924) (314.6836, 602.548) (315.017, 602.711) (315.2047, 602.711) knots 0 0 0 1 2 2 2
  spline S987 degree 2 poles (315.2047, 602.711) (315.5407, 602.711) (315.921, 602.2664) (315.921, 601.844) knots 0 0 0 1 2 2 2
  line L998 (315.921, 601.844) -> (315.921, 600.3596)
  spline S988 degree 2 poles (317.4549, 600.3077) (316.9066, 600.3077) (316.3039, 600.9227) (316.3039, 601.4908) knots 0 0 0 1 2 2 2
  spline S989 degree 2 poles (316.3039, 601.4908) (316.3039, 602.0491) (316.8893, 602.711) (317.3611, 602.711) knots 0 0 0 1 2 2 2
  spline S990 degree 2 poles (317.3611, 602.711) (317.5735, 602.711) (317.902, 602.5875) (318.023, 602.4566) knots 0 0 0 1 2 2 2
  spline S991 degree 2 poles (318.023, 602.4566) (318.1465, 602.3257) (318.2774, 601.9478) (318.2774, 601.6736) knots 0 0 0 1 2 2 2
  line L999 (318.2774, 601.6736) -> (318.2774, 601.4637)
  line L1000 (318.2774, 601.4637) -> (316.6941, 601.4637)
  spline S992 degree 2 poles (316.6941, 601.4637) (316.6941, 601.066) (317.0943, 600.6436) (317.45, 600.6436) knots 0 0 0 1 2 2 2
  spline S993 degree 2 poles (317.45, 600.6436) (317.5759, 600.6436) (317.8205, 600.7004) (317.9193, 600.7449) knots 0 0 0 1 2 2 2
  spline S994 degree 2 poles (317.9193, 600.7449) (318.023, 600.7943) (318.1663, 600.8807) (318.2132, 600.9203) knots 0 0 0 1 2 2 2
  line L1001 (318.2132, 600.9203) -> (318.2354, 600.9203)
  line L1002 (318.2354, 600.9203) -> (318.2354, 600.5004)
  spline S995 degree 2 poles (318.2354, 600.5004) (318.1687, 600.4732) (317.9662, 600.3941) (317.8872, 600.3719) knots 0 0 0 1 2 2 2
  spline S996 degree 2 poles (317.8872, 600.3719) (317.776, 600.3398) (317.5932, 600.3077) (317.4549, 600.3077) knots 0 0 0 1 2 2 2
  spline S997 degree 2 poles (317.902, 601.7576) (317.897, 601.9132) (317.8328, 602.1404) (317.7711, 602.217) knots 0 0 0 1 2 2 2
  spline S998 degree 2 poles (317.7711, 602.217) (317.7044, 602.3035) (317.4944, 602.3949) (317.3388, 602.3949) knots 0 0 0 1 2 2 2
  spline S999 degree 2 poles (317.3388, 602.3949) (317.1857, 602.3949) (316.9708, 602.3035) (316.8819, 602.2145) knots 0 0 0 1 2 2 2
  spline S1000 degree 2 poles (316.8819, 602.2145) (316.7954, 602.1232) (316.7065, 601.9033) (316.6941, 601.7576) knots 0 0 0 1 2 2 2
  line L1003 (316.6941, 601.7576) -> (317.902, 601.7576)
  spline S1001 degree 2 poles (319.2852, 600.3052) (319.0555, 600.3052) (318.6578, 600.4287) (318.5269, 600.4979) knots 0 0 0 1 2 2 2
  line L1004 (318.5269, 600.4979) -> (318.5269, 600.9301)
  line L1005 (318.5269, 600.9301) -> (318.5467, 600.9301)
  spline S1002 degree 2 poles (318.5467, 600.9301) (318.5961, 600.8906) (318.7294, 600.7968) (318.8406, 600.7449) knots 0 0 0 1 2 2 2
  spline S1003 degree 2 poles (318.8406, 600.7449) (318.9369, 600.698) (319.174, 600.6288) (319.3, 600.6288) knots 0 0 0 1 2 2 2
  spline S1004 degree 2 poles (319.3, 600.6288) (319.3914, 600.6288) (319.6014, 600.6708) (319.6508, 600.7054) knots 0 0 0 1 2 2 2
  spline S1005 degree 2 poles (319.6508, 600.7054) (319.7224, 600.7523) (319.7866, 600.8585) (319.7866, 600.9672) knots 0 0 0 1 2 2 2
  spline S1006 degree 2 poles (319.7866, 600.9672) (319.7866, 601.103) (319.6384, 601.2438) (319.4482, 601.2908) knots 0 0 0 1 2 2 2
  spline S1007 degree 2 poles (319.4482, 601.2908) (319.3741, 601.3081) (319.137, 601.3575) (319.0357, 601.3846) knots 0 0 0 1 2 2 2
  spline S1008 degree 2 poles (319.0357, 601.3846) (318.7739, 601.4612) (318.5368, 601.7774) (318.5368, 602.0021) knots 0 0 0 1 2 2 2
  spline S1009 degree 2 poles (318.5368, 602.0021) (318.5368, 602.3133) (319.0036, 602.7011) (319.3889, 602.7011) knots 0 0 0 1 2 2 2
  spline S1010 degree 2 poles (319.3889, 602.7011) (319.5791, 602.7011) (319.9645, 602.6073) (320.0954, 602.5356) knots 0 0 0 1 2 2 2
  line L1006 (320.0954, 602.5356) -> (320.0954, 602.1232)
  line L1007 (320.0954, 602.1232) -> (320.0756, 602.1232)
  spline S1011 degree 2 poles (320.0756, 602.1232) (319.9274, 602.2417) (319.5668, 602.3776) (319.3815, 602.3776) knots 0 0 0 1 2 2 2
  spline S1012 degree 2 poles (319.3815, 602.3776) (319.1913, 602.3776) (318.9295, 602.217) (318.9295, 602.0565) knots 0 0 0 1 2 2 2
  spline S1013 degree 2 poles (318.9295, 602.0565) (318.9295, 601.9107) (319.0851, 601.7699) (319.258, 601.7255) knots 0 0 0 1 2 2 2
  spline S1014 degree 2 poles (319.258, 601.7255) (319.342, 601.7033) (319.5544, 601.6588) (319.6705, 601.6316) knots 0 0 0 1 2 2 2
  spline S1015 degree 2 poles (319.6705, 601.6316) (319.9225, 601.5674) (320.1793, 601.2735) (320.1793, 601.0191) knots 0 0 0 1 2 2 2
  spline S1016 degree 2 poles (320.1793, 601.0191) (320.1793, 600.8709) (320.0633, 600.609) (319.9496, 600.5127) knots 0 0 0 1 2 2 2
  spline S1017 degree 2 poles (319.9496, 600.5127) (319.8286, 600.4114) (319.5198, 600.3052) (319.2852, 600.3052) knots 0 0 0 1 2 2 2
  spline S1018 degree 2 poles (321.155, 600.3052) (320.9253, 600.3052) (320.5276, 600.4287) (320.3967, 600.4979) knots 0 0 0 1 2 2 2
  line L1008 (320.3967, 600.4979) -> (320.3967, 600.9301)
  line L1009 (320.3967, 600.9301) -> (320.4165, 600.9301)
  spline S1019 degree 2 poles (320.4165, 600.9301) (320.4659, 600.8906) (320.5992, 600.7968) (320.7104, 600.7449) knots 0 0 0 1 2 2 2
  spline S1020 degree 2 poles (320.7104, 600.7449) (320.8067, 600.698) (321.0438, 600.6288) (321.1698, 600.6288) knots 0 0 0 1 2 2 2
  spline S1021 degree 2 poles (321.1698, 600.6288) (321.2612, 600.6288) (321.4712, 600.6708) (321.5206, 600.7054) knots 0 0 0 1 2 2 2
  spline S1022 degree 2 poles (321.5206, 600.7054) (321.5922, 600.7523) (321.6564, 600.8585) (321.6564, 600.9672) knots 0 0 0 1 2 2 2
  spline S1023 degree 2 poles (321.6564, 600.9672) (321.6564, 601.103) (321.5082, 601.2438) (321.318, 601.2908) knots 0 0 0 1 2 2 2
  spline S1024 degree 2 poles (321.318, 601.2908) (321.2439, 601.3081) (321.0068, 601.3575) (320.9055, 601.3846) knots 0 0 0 1 2 2 2
  spline S1025 degree 2 poles (320.9055, 601.3846) (320.6437, 601.4612) (320.4066, 601.7774) (320.4066, 602.0021) knots 0 0 0 1 2 2 2
  spline S1026 degree 2 poles (320.4066, 602.0021) (320.4066, 602.3133) (320.8734, 602.7011) (321.2587, 602.7011) knots 0 0 0 1 2 2 2
  spline S1027 degree 2 poles (321.2587, 602.7011) (321.4489, 602.7011) (321.8343, 602.6073) (321.9652, 602.5356) knots 0 0 0 1 2 2 2
  line L1010 (321.9652, 602.5356) -> (321.9652, 602.1232)
  line L1011 (321.9652, 602.1232) -> (321.9454, 602.1232)
  spline S1028 degree 2 poles (321.9454, 602.1232) (321.7972, 602.2417) (321.4366, 602.3776) (321.2513, 602.3776) knots 0 0 0 1 2 2 2
  spline S1029 degree 2 poles (321.2513, 602.3776) (321.0611, 602.3776) (320.7993, 602.217) (320.7993, 602.0565) knots 0 0 0 1 2 2 2
  spline S1030 degree 2 poles (320.7993, 602.0565) (320.7993, 601.9107) (320.9549, 601.7699) (321.1278, 601.7255) knots 0 0 0 1 2 2 2
  spline S1031 degree 2 poles (321.1278, 601.7255) (321.2118, 601.7033) (321.4242, 601.6588) (321.5403, 601.6316) knots 0 0 0 1 2 2 2
  spline S1032 degree 2 poles (321.5403, 601.6316) (321.7923, 601.5674) (322.0491, 601.2735) (322.0491, 601.0191) knots 0 0 0 1 2 2 2
  spline S1033 degree 2 poles (322.0491, 601.0191) (322.0491, 600.8709) (321.9331, 600.609) (321.8194, 600.5127) knots 0 0 0 1 2 2 2
  spline S1034 degree 2 poles (321.8194, 600.5127) (321.6984, 600.4114) (321.3896, 600.3052) (321.155, 600.3052) knots 0 0 0 1 2 2 2
  point P0 (0, 0)
  constraints: 2 other
extrude "Extrusion5" add sketch "Sketch6" along normal blind 0.254
body "Solid1"
